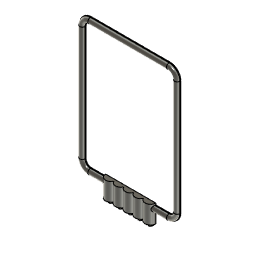
SolderingStation_DisplayFrame (Autodesk Fusion 360 design; units mm, degrees)
Autodesk Fusion 360 part; units mm, degrees
sketch "Sketch1" plane through (0, 0, 0) normal (0, 1, 0) x (1, 0, 0)
  line L0 (21.9, -34.9) -> (-21.9, -34.9)
  line L1 (-24.9, -31.9) -> (-24.9, 31.9)
  line L2 (-21.9, 34.9) -> (21.9, 34.9)
  line L3 (24.9, 31.9) -> (24.9, -31.9)
  line L4 (24.9, -34.9) -> (-24.9, 34.9) construction
  line L5 (-24.9, -34.9) -> (24.9, 34.9) construction
  arc A0 (-24.9, -31.9) -> (-21.9, -34.9) centre (-21.9, -31.9) ccw
  arc A1 (21.9, -34.9) -> (24.9, -31.9) centre (21.9, -31.9) ccw
  arc A2 (-21.9, 34.9) -> (-24.9, 31.9) centre (-21.9, 31.9) ccw
  arc A3 (24.9, 31.9) -> (21.9, 34.9) centre (21.9, 31.9) ccw
  line L6 (27.9, 31.9) -> (27.9, -31.9)
  arc A4 (21.9, -37.9) -> (27.9, -31.9) centre (21.9, -31.9) ccw
  line L7 (21.9, -37.9) -> (-21.9, -37.9)
  arc A5 (-27.9, -31.9) -> (-21.9, -37.9) centre (-21.9, -31.9) ccw
  line L8 (-27.9, -31.9) -> (-27.9, 31.9)
  arc A6 (-21.9, 37.9) -> (-27.9, 31.9) centre (-21.9, 31.9) ccw
  line L9 (-21.9, 37.9) -> (21.9, 37.9)
  arc A7 (27.9, 31.9) -> (21.9, 37.9) centre (21.9, 31.9) ccw
  dimension "d1" = 49.8
  dimension "d2" = 69.8
  dimension "d3" = -3
  dimension "d6" = 3
  dimension "d7" = 3
  dimension "d8" = 3
  dimension "d9" = 3
  constraint horizontal L0
  constraint perpendicular L0 L1
  constraint parallel L0 L2
  constraint parallel L1 L3
  constraint coincident L4 origin
  constraint coincident L5 origin
  constraint coincident L5.start L1
  constraint coincident L5.start L0
  constraint tangent L1 A0
  constraint tangent L0 A0
  constraint coincident L4.start L0
  constraint coincident L4.start L3
  constraint tangent L0 A1
  constraint tangent L3 A1
  constraint coincident L4.end L2
  constraint coincident L4.end L1
  constraint tangent L2 A2
  constraint tangent L1 A2
  constraint coincident L5.end L2
  constraint coincident L5.end L3
  constraint tangent L2 A3
  constraint tangent L3 A3
  measures "d1" distance of L4.end L5.end
  measures "d2" distance of L5.start L4.end
  measures "d6" radius of A0
  measures "d7" radius of A1
  measures "d8" radius of A2
  measures "d9" radius of A3
extrude "Extrude1" add sketch "Sketch1" along normal blind 2
fillet "Fillet1" radius 1.5 16 edges at (0, 0, -34.9) (24.0213, 0, -34.0213) (24.9, 0, 0) (24.0213, 0, 34.0213) (0, 0, 34.9) (-24.0213, 0, 34.0213) (-24.9, 0, 0) (-24.0213, 0, -34.0213) (-26.1426, 0, -36.1426) (-27.9, 0, 0) (-26.1426, 0, 36.1426) (0, 0, 37.9) (26.1426, 0, 36.1426) (27.9, 0, 0) (26.1426, 0, -36.1426) (0, 0, -37.9)
ref_plane "WorkPlane1" through (0, 0, -38) normal (0, 0, 1) x (1, 0, 0)
sketch "Sketch3" plane through (0, 0, -38) normal (0, 0, 1) x (1, 0, 0)
  line L0 (0, 0) -> (0, 2) construction
  circle A0 centre (0, 2) radius 3
  circle A1 centre (5.5, 2) radius 3
  circle A2 centre (11, 2) radius 3
  circle A3 centre (-5.5, 2) radius 3
  circle A4 centre (-11, 2) radius 3
  line L1 (0, 2) -> (-14, 2)
  line L2 (0, 2) -> (14, 2)
  dimension "d34" = 6
  dimension "d35" = 6
  dimension "d36" = 6
  dimension "d38" = 6
  dimension "d39" = 6
  constraint coincident L0.start origin
  constraint vertical L0
  constraint coincident L0.end A0.centre
  constraint coincident A4 L1.end
  constraint perpendicular L0 L1
  constraint coincident A2 L2.end
  constraint perpendicular L0 L2
  constraint coincident A1.centre L2
  constraint coincident A3.centre L1
  measures "d34" diameter of A0
  measures "d35" diameter of A1
  measures "d36" diameter of A2
  measures "d38" diameter of A3
  measures "d39" diameter of A4
extrude "Extrude3" add sketch "Sketch3" along normal blind 4 and the other way blind 8 contours A0 A1 A2 L2 | A0 A1 L2 | A0 A1 A3 L1 L2 | A1 A2 L2 | A0 A3 A4 L1 | A0 A3 L1 | A1 A2 L2 | A3 A4 L1 | A3 A4 L1 picked at (5.5, 0.7268) picked at (2.676, 1.8634) picked at (1.6348, 1.0843) picked at (8.176, 1.8634) picked at (-5.5, 0.7268) picked at (-2.824, 1.8634) picked at (12.1564, 1.8568) picked at (-12.1564, 1.8568) picked at (-8.324, 1.8634)
chamfer "Chamfer2" distance 2 angle 45 5 edges at (-11.6124, -0.9368, -46) (-5.5, -1, -46) (0, -1, -46) (5.5, -1, -46) (11.6124, -0.9368, -46)
sketch "Sketch5" plane through (0, 0, -34) normal (0, 0, 1) x (-1, 0, 0)
  line L0 (-14, -2) -> (14, -2)
  arc A0 (14, -2) -> (8.25, -0.801) centre (11, -2) ccw
  arc A1 (8.25, -0.801) -> (2.75, -0.801) centre (5.5, -2) ccw
  arc A2 (2.75, -0.801) -> (-2.75, -0.801) centre (0, -2) ccw
  arc A3 (-2.75, -0.801) -> (-8.25, -0.801) centre (-5.5, -2) ccw
  arc A4 (-8.25, -0.801) -> (-14, -2) centre (-11, -2) ccw
  line L1 (0, 0) -> (0, -2) construction
  circle A5 centre (0, -2) radius 3
  circle A6 centre (5.5, -2) radius 3
  circle A7 centre (11, -2) radius 3
  circle A8 centre (-5.5, -2) radius 3
  circle A9 centre (-11, -2) radius 3
  line L2 (11, -2) -> (11, 1) construction
  line L3 (-11, -2) -> (-11, 1) construction
  line L4 (11, 1) -> (-11, 1)
  constraint coincident L1.start origin
  constraint coincident A2.centre L1.end
  constraint concentric A1 A6
  constraint concentric A0 A7
  constraint concentric A3 A8
  constraint concentric A4 A9
  constraint vertical L2
  constraint coincident A0.centre A7.centre
  constraint vertical L3
  constraint coincident A4.centre A9.centre
  constraint tangent A4 L4
extrude "Extrude4" cut sketch "Sketch5" against normal blind 10 contours A0 A1 A6 A7 L4 | A1 A2 A5 A6 L4 | A2 A3 A5 A8 L4 | A3 A4 A8 A9 L4
